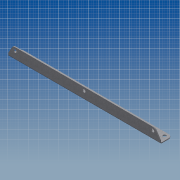
# Autodesk Inventor part: J009835
Saved by Autodesk Inventor 2020.3 (Build 243373000, 373)
## iProperties
RuleStatus: InUse
AfterDocSave0: file://Part Number Cleaner
Created: 2021-03-26
Material: STAINLESS STEEL, 316
Catalog Web Link: https://www.janelia.org/
Vendor: HHMI: JRC - ID&F
Document SubType Name: Sheet Metal
Designer: talbotj
Density: 8 g/cm^3
Sheet Metal Rule: Default
Appearance: Metal-Steel (Stainless, Brushed)
Flat Pattern Width: 2.39863 cm
Flat Pattern Length: 16.129 cm
Flat Pattern Area: 38.6875 cm^2
Sheet Metal Width: 0.944 in
Sheet Metal Length: 6.350 in
Sheet Metal Area: 5.997 in^2
Part Number: J009835
Description: N/A
Project: N/A
DESIGN DEPARTMENT: HHMI: JRC - ID&F
SPECIAL FINISH: N/A
LAB/DEPT: VIVARIUM (SHARED RESOURCES)
REQUESTING SCIENTIST: COX, JAMES
SURFACE ROUGHNESS: N/A
Thickness: 0.036 in
ALTERED ITEM PART NUMBER: N/A
ALTERED ITEM VENDOR: N/A
ALTERED ITEM DESCRIPTION: N/A
PART NUMBER - LEGACY: N/A
Author: talbotj
Revision Number: -
Autodesk Inventor part; units mm, degrees
ref_plane "YZ Plane" through (0, 0, 0) normal (1, 0, 0) x (0, 1, 0)
ref_plane "XZ Plane" through (0, 0, 0) normal (0, 1, 0) x (-1, 0, 0)
ref_plane "XY Plane" through (0, 0, 0) normal (0, 0, 1) x (1, 0, 0)
sketch "Sketch1" plane through (0, 0, 0) normal (0, 1, 0) x (-1, 0, 0)
  line L0 (-80.645, 0) -> (80.645, 0)
  line L1 (80.645, 0) -> (80.645, 12.7)
  line L2 (80.645, 12.7) -> (-80.645, 12.7)
  line L3 (-80.645, 12.7) -> (-80.645, 0)
  line L4 (-80.645, 0) -> (80.645, 12.7) construction
  line L5 (80.645, 0) -> (-80.645, 12.7) construction
  point P0 (0, 0)
  point P1 (0, 6.35)
  point P2 (0, 0)
  dimension "d0" = 12.7
  dimension "d1" = 161.29
  measures "d0" distance of L0.end L1.end
  measures "d1" distance of L1.end L2.end
extrude "Plate1" add sketch "Sketch1" along normal blind 0.9144
sketch "Sketch2" plane through (80.645, 0.0479, 11.7869) normal (0, -0.052336, 0.9986295) x (1, 0, 0)
  line L0 (-161.29, 0) -> (0, 0)
  line L1 (0, 0) -> (0, 12.7)
  line L2 (0, 12.7) -> (-161.29, 12.7)
  line L3 (-161.29, 12.7) -> (-161.29, 0)
  constraints: 6 end point, 1 horizontal, 1 perpendicular, 1 vertical
edge flange "Flange1" height 12.7 angle 87 thickness 0.9144 bend radius 0.762 thickness toward (0, -0.052336, 0.9986295) relief tear relief width 0.9144 relief depth 0.4572 edges at (0, 0.9144, 12.7) wall of the first edge with corners at (-80.645, 0.0479, 11.7869) (80.645, 0.0479, 11.7869) (80.645, 12.7305, 12.4515) (-80.645, 12.7305, 12.4515)
bend "Bend1"
corner "Corner1"
sketch "Sketch3" plane through (0, 0.9144, 0) normal (0, 1, 0) x (1, 0, 0)
  line L0 (76.2, -3.81) -> (-76.2, -3.81) construction
  line L1 (-80.645, 0) -> (80.645, 0) construction
  point P0 (0, 0)
  point P1 (0, -3.81)
  point P2 (0, -3.81)
  point P3 (0, 0)
  dimension "d13" = 152.4
  dimension "d14" = 3.81
  constraints: 2 end point, 2 midpoint, 1 coincident, 1 horizontal, 1 vertical alignment
  measures "d13" distance of L0.start L0.end
  measures "d14" distance between parallel lines of L1 L0
hole "Hole1" at (76.2, 0.9144, 3.81) at (0, 0.9144, 3.81) at (-76.2, 0.9144, 3.81) direction (0, -1, 0) diameter 3.2512 end through all
sketch "Sketch4" plane through (80.645, 12.7305, 12.4515) normal (0, 0.052336, -0.9986295) x (-1, 0, 0)
  line L0 (7.62, -3.81) -> (153.67, -3.81) construction
  line L1 (161.29, 0) -> (0, 0) construction
  point P0 (80.645, -13.3647)
  point P1 (80.645, -3.81)
  point P2 (80.645, -3.81)
  dimension "d22" = 146.05
  dimension "d23" = 3.81
  constraints: 2 end point, 1 coincident, 1 horizontal, 1 midpoint, 1 vertical alignment
  measures "d22" distance of L0.start L0.end
  measures "d23" distance between parallel lines of L0 L1
hole "Hole2" at (73.025, 8.9257, 12.2521) at (0, 8.9257, 12.2521) at (-73.025, 8.9257, 12.2521) direction (0, -0.052336, 0.9986295) diameter 3.2512 end through all
chamfer "Corner Chamfer1" distance 5.588 angle 60 2 edges at (-80.645, 12.7065, 12.9081) (80.645, 12.7065, 12.9081) measured on face at (-26.8817, 12.6985, 13.0603)
fillet "Corner Round1" radius 3.81 6 edges at (80.645, 0.4572, 0) (-80.645, 0.4572, 0) (-75.057, 12.7065, 12.9081) (75.057, 12.7065, 12.9081) (-80.645, 3.0411, 12.4015) (80.645, 3.0411, 12.4015)
equation "\"d20\" = Thickness"
equation "\"d29\" = Thickness"
equation "\"d2\" = Thickness"
equation "\"d3\" = BendReliefWidth"
equation "\"d4\" = BendReliefDepth"
equation "\"d5\" = MinimumRemnant"
equation "\"d6\" = TransitionRadius"
equation "\"d9\" = BendRadius"
equation "\"d10\" = CornerReliefSize"
equation "\"d11\" = GapSize"
equation "\"d12\" = JacobiRadiusSize"
equation "\"BendReliefWidth\" = Thickness"
equation "\"BendReliefDepth\" = 0.5 * Thickness"
equation "\"CornerReliefSize\" = 4 * Thickness"
equation "\"MinimumRemnant\" = 2 * Thickness"
equation "\"TransitionRadius\" = BendRadius"
equation "\"JacobiRadiusSize\" = BendRadius"
equation "\"GapSize\" = Thickness"
equation "\"Thickness\" = 0.9144"
equation "\"BendRadius\" = 0.762"
body "Solid1"
